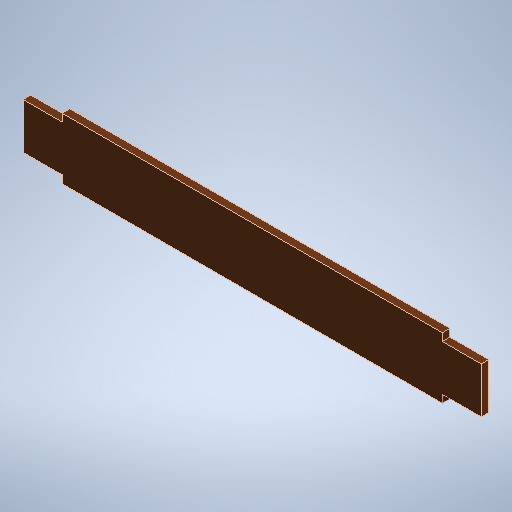
# Autodesk Inventor part: Base Leg V2
Saved by Autodesk Inventor 2025.4 (Build 294407000, 407)
## iProperties
Created: 2026-03-23
Part Number: Base Leg V2
Material: Generic
Document SubType Name: Sheet Metal
Designer: lenovo
Density: 1 g/cm^3
Sheet Metal Rule: Default_mm
Appearance: Default(1)
Author: lenovo
Autodesk Inventor part; units mm, degrees
ref_plane "YZ Plane" through (0, 0, 0) normal (1, 0, 0) x (0, 1, 0)
ref_plane "XZ Plane" through (0, 0, 0) normal (0, 1, 0) x (-1, 0, 0)
ref_plane "XY Plane" through (0, 0, 0) normal (0, 0, 1) x (1, 0, 0)
sketch "Sketch1" plane through (0, 0, 0) normal (0, 0, 1) x (1, 0, 0)
  line L0 (-150, -15) -> (150, -15)
  line L1 (150, -15) -> (150, 15)
  line L2 (150, 15) -> (-150, 15)
  line L3 (-150, 15) -> (-150, -15)
  line L4 (-150, -15) -> (150, 15) construction
  line L5 (150, -15) -> (-150, 15) construction
  line L6 (-124.5, 20) -> (124.5, 20)
  line L7 (124.5, 20) -> (124.5, 15)
  line L8 (124.5, 15) -> (-124.5, 15)
  line L9 (-124.5, 15) -> (-124.5, 20)
  line L10 (-124.5, 20) -> (124.5, 15) construction
  line L11 (124.5, 20) -> (-124.5, 15) construction
  line L12 (-150, 0) -> (150, 0)
  line L13 (-124.5, -20) -> (124.5, -20)
  line L14 (124.5, -20) -> (124.5, -15)
  line L15 (124.5, -15) -> (-124.5, -15)
  line L16 (-124.5, -15) -> (-124.5, -20)
  line L17 (-124.5, -20) -> (124.5, -15) construction
  line L18 (124.5, -20) -> (-124.5, -15) construction
  point P0 (0, 0)
  point P1 (0, 0)
  point P2 (0, 17.5)
  point P3 (0, 15)
  point P4 (-77.3047, 14.0744)
  point P5 (81.6953, 14.0744)
  point P6 (0, -15)
  point P7 (0, -17.5)
  dimension "d0" = 5
  dimension "d1" = 30
  dimension "d2" = 300
  dimension "d3" = 249
  measures "d0" distance of L8.end L6.start
  measures "d1" distance of L2.end L0.start
  measures "d2" distance of L0.start L0.end
  measures "d3" distance of L6.start L6.end
extrude "Plate1" add sketch "Sketch1" along normal blind 5
equation "\"d4\" = Thickness"
equation "\"BendRadius\" = Thickness"
equation "\"BendReliefWidth\" = Thickness"
equation "\"BendReliefDepth\" = 0.5 * Thickness"
equation "\"TransitionRadius\" = BendRadius"
equation "\"JacobiRadiusSize\" = BendRadius"
equation "\"GapSize\" = Thickness"
equation "\"Thickness\" = 5"
body "Solid1"
